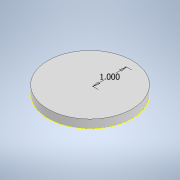
# Autodesk Inventor part: Blue Alliance Marker
Saved by Autodesk Inventor 2020 (Build 240168000, 168)
## iProperties
Created: 2020-01-13
Part Number: Blue Alliance Marker
Material: Generic
Document SubType Name: Modeling
Designer: maple
Density: 1 g/cm^3
Appearance: Default
Author: maple
Autodesk Inventor part; units mm, degrees
ref_plane "YZ Plane" through (0, 0, 0) normal (1, 0, 0) x (0, 1, 0)
ref_plane "XZ Plane" through (0, 0, 0) normal (0, 1, 0) x (-1, 0, 0)
ref_plane "XY Plane" through (0, 0, 0) normal (0, 0, 1) x (1, 0, 0)
sketch "Sketch1" plane through (0, 0, 0) normal (0, 1, 0) x (-1, 0, 0)
  circle A0 centre (0, 0) radius 31.75
  dimension "d0" = 63.5
  constraints: 1 centre point, 1 coincident
  measures "d0" diameter of A0
extrude "Extrusion1" add sketch "Sketch1" along normal blind 6.35
sketch "Sketch2" plane through (0, 0, 0) normal (0, -1, 0) x (1, 0, 0)
  line L0 (-4.9346, 27.7606) -> (4.7207, 27.7606) construction
  line L1 (4.7207, 27.7606) -> (4.7207, 24.6484) construction
  line L2 (4.7207, 24.6484) -> (-4.9346, 24.6484) construction
  line L3 (-4.9346, 24.6484) -> (-4.9346, 27.7606) construction
  spline S0 degree 2 poles (-2.5584, 25.6488) (-2.5584, 25.4215) (-2.7313, 25.0733) (-2.8746, 24.9596) knots 0 0 0 1 2 2 2
  spline S1 degree 2 poles (-2.8746, 24.9596) (-3.0475, 24.8263) (-3.4402, 24.7126) (-3.7514, 24.7126) knots 0 0 0 1 2 2 2
  line L4 (-3.7514, 24.7126) -> (-4.6258, 24.7126)
  line L5 (-4.6258, 24.7126) -> (-4.6258, 27.7606)
  line L6 (-4.6258, 27.7606) -> (-3.8181, 27.7606)
  spline S2 degree 2 poles (-3.8181, 27.7606) (-3.4921, 27.7606) (-3.166, 27.7187) (-3.0178, 27.6371) knots 0 0 0 1 2 2 2
  spline S3 degree 2 poles (-3.0178, 27.6371) (-2.8524, 27.5507) (-2.7017, 27.2666) (-2.7017, 27.074) knots 0 0 0 1 2 2 2
  spline S4 degree 2 poles (-2.7017, 27.074) (-2.7017, 26.8591) (-2.9289, 26.5182) (-3.129, 26.4219) knots 0 0 0 1 2 2 2
  line L7 (-3.129, 26.4219) -> (-3.129, 26.4071)
  spline S5 degree 2 poles (-3.129, 26.4071) (-2.8573, 26.333) (-2.5584, 25.9402) (-2.5584, 25.6488) knots 0 0 0 1 2 2 2
  spline S6 degree 2 poles (-2.9808, 25.6315) (-2.9808, 25.8044) (-3.0796, 26.0267) (-3.2278, 26.1057) knots 0 0 0 1 2 2 2
  spline S7 degree 2 poles (-3.2278, 26.1057) (-3.3241, 26.1551) (-3.5514, 26.1848) (-3.7613, 26.1848) knots 0 0 0 1 2 2 2
  line L8 (-3.7613, 26.1848) -> (-4.2207, 26.1848)
  line L9 (-4.2207, 26.1848) -> (-4.2207, 25.0584)
  line L10 (-4.2207, 25.0584) -> (-3.8922, 25.0584)
  spline S8 degree 2 poles (-3.8922, 25.0584) (-3.6255, 25.0584) (-3.3192, 25.1078) (-3.2006, 25.1869) knots 0 0 0 1 2 2 2
  spline S9 degree 2 poles (-3.2006, 25.1869) (-3.087, 25.2684) (-2.9808, 25.4709) (-2.9808, 25.6315) knots 0 0 0 1 2 2 2
  spline S10 degree 2 poles (-3.1241, 27.0172) (-3.1241, 27.1258) (-3.1982, 27.2889) (-3.2797, 27.3358) knots 0 0 0 1 2 2 2
  spline S11 degree 2 poles (-3.2797, 27.3358) (-3.3785, 27.3901) (-3.6181, 27.4148) (-3.8329, 27.4148) knots 0 0 0 1 2 2 2
  line L11 (-3.8329, 27.4148) -> (-4.2207, 27.4148)
  line L12 (-4.2207, 27.4148) -> (-4.2207, 26.5232)
  line L13 (-4.2207, 26.5232) -> (-3.7613, 26.5232)
  spline S12 degree 2 poles (-3.7613, 26.5232) (-3.5711, 26.5232) (-3.3908, 26.5627) (-3.2945, 26.6244) knots 0 0 0 1 2 2 2
  spline S13 degree 2 poles (-3.2945, 26.6244) (-3.2006, 26.6837) (-3.1241, 26.8739) (-3.1241, 27.0172) knots 0 0 0 1 2 2 2
  line L14 (-0.3897, 24.7126) -> (-2.1558, 24.7126)
  line L15 (-2.1558, 24.7126) -> (-2.1558, 27.7606)
  line L16 (-2.1558, 27.7606) -> (-1.7507, 27.7606)
  line L17 (-1.7507, 27.7606) -> (-1.7507, 25.0733)
  line L18 (-1.7507, 25.0733) -> (-0.3897, 25.0733)
  line L19 (-0.3897, 25.0733) -> (-0.3897, 24.7126)
  spline S14 degree 2 poles (0.9935, 24.6484) (0.7242, 24.6484) (0.3241, 24.7892) (0.1833, 24.93) knots 0 0 0 1 2 2 2
  spline S15 degree 2 poles (0.1833, 24.93) (0.0227, 25.0881) (-0.1082, 25.5327) (-0.1082, 25.8587) knots 0 0 0 1 2 2 2
  line L20 (-0.1082, 25.8587) -> (-0.1082, 27.7606)
  line L21 (-0.1082, 27.7606) -> (0.2969, 27.7606)
  line L22 (0.2969, 27.7606) -> (0.2969, 25.8587)
  spline S16 degree 2 poles (0.2969, 25.8587) (0.2969, 25.6463) (0.3513, 25.3598) (0.4278, 25.2437) knots 0 0 0 1 2 2 2
  spline S17 degree 2 poles (0.4278, 25.2437) (0.5093, 25.1202) (0.7909, 24.9942) (0.9935, 24.9942) knots 0 0 0 1 2 2 2
  spline S18 degree 2 poles (0.9935, 24.9942) (1.1837, 24.9942) (1.4801, 25.1202) (1.5616, 25.2437) knots 0 0 0 1 2 2 2
  spline S19 degree 2 poles (1.5616, 25.2437) (1.6381, 25.3598) (1.6925, 25.6438) (1.6925, 25.8489) knots 0 0 0 1 2 2 2
  line L23 (1.6925, 25.8489) -> (1.6925, 27.7606)
  line L24 (1.6925, 27.7606) -> (2.0976, 27.7606)
  line L25 (2.0976, 27.7606) -> (2.0976, 25.8587)
  spline S20 degree 2 poles (2.0976, 25.8587) (2.0976, 25.5401) (1.9691, 25.0856) (1.8061, 24.93) knots 0 0 0 1 2 2 2
  spline S21 degree 2 poles (1.8061, 24.93) (1.6604, 24.7867) (1.275, 24.6484) (0.9935, 24.6484) knots 0 0 0 1 2 2 2
  line L26 (2.678, 24.7126) -> (2.678, 27.7606)
  line L27 (2.678, 27.7606) -> (4.5849, 27.7606)
  line L28 (4.5849, 27.7606) -> (4.5849, 27.4)
  line L29 (4.5849, 27.4) -> (3.0831, 27.4)
  line L30 (3.0831, 27.4) -> (3.0831, 26.5652)
  line L31 (3.0831, 26.5652) -> (4.4836, 26.5652)
  line L32 (4.4836, 26.5652) -> (4.4836, 26.2045)
  line L33 (4.4836, 26.2045) -> (3.0831, 26.2045)
  line L34 (3.0831, 26.2045) -> (3.0831, 25.0733)
  line L35 (3.0831, 25.0733) -> (4.5849, 25.0733)
  line L36 (4.5849, 25.0733) -> (4.5849, 24.7126)
  line L37 (4.5849, 24.7126) -> (2.678, 24.7126)
  point P0 (0, 0)
  constraints: 2 other
emboss "Emboss1" sketch "Sketch2" operation add depth 0.508 direction (0, 1, 0)
sketch "Sketch3" plane through (0, 0, 0) normal (0, -1, 0) x (1, 0, 0)
  circle A0 centre (0, 0) radius 31.75 projected
  line L0 (0, -31.75) -> (0, -6.35)
  dimension "d5" = 25.4
  constraints: 2 end point, 1 vertical, 1 vertical alignment, 1 other
  measures "d5" distance of L0.start L0.end
body "Solid1"
